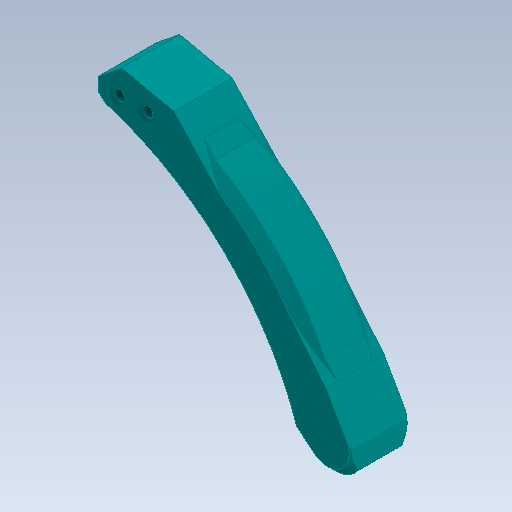
# Autodesk Inventor part: Tarsus
Saved by Autodesk Inventor 2020 (Build 240168000, 168)
## iProperties
Created: 2020-09-15
Part Number: Tarsus
Material: Generic
Document SubType Name: Modeling
Designer: Turing
Density: 1 g/cm^3
Appearance: Gray
Mass: 22.7557 g
Surface Area: 61.6652 cm^2
Volume: 22.7557 cm^3
Author: Turing
Autodesk Inventor part; units mm, degrees
ref_plane "YZ Plane" through (0, 0, 0) normal (1, 0, 0) x (0, 1, 0)
ref_plane "XZ Plane" through (0, 0, 0) normal (0, 1, 0) x (-1, 0, 0)
ref_plane "XY Plane" through (0, 0, 0) normal (0, 0, 1) x (1, 0, 0)
sketch "Sketch1" plane through (0, 0, 0) normal (0, 0, 1) x (1, 0, 0)
  circle A0 centre (0, 0) radius 1.5
  line L0 (0, 0) -> (8, 0)
  circle A1 centre (8, 0) radius 1.5
  line L1 (8, 0) -> (15.5, 0)
  line L2 (15.5, 0) -> (15.5, 4)
  line L3 (15.5, 0) -> (15.5, -4)
  line L4 (15.5, 4) -> (0.8426, 7.1878)
  line L5 (15.5, -4) -> (0.8886, -7.3921)
  line L6 (0, 0) -> (-8, 0)
  line L7 (0.8886, -7.3921) -> (-8, 0)
  line L8 (-8, 0) -> (0.8426, 7.1878)
  dimension "d0" = 3
  dimension "d1" = 8
  dimension "d2" = 3
  dimension "d3" = 7.5
  dimension "d4" = 4
  dimension "d5" = 4
  dimension "d6" = 102.27
  dimension "d7" = 103.07
  dimension "d8" = 15
  dimension "d9" = 15
  dimension "d10" = 8
  constraints: 18 end point, 3 horizontal, 2 centre point, 2 coincident, 2 vertical
  measures "d0" diameter of A0
  measures "d1" distance of L0.start L0.end
  measures "d2" diameter of A1
  measures "d3" distance of L1.start L1.end
  measures "d4" distance of L1.end L2.end
  measures "d5" distance of L1.end L3.end
  measures "d6" angle of L2 L4
  measures "d7" angle of L3 L5
  measures "d8" distance of L3.end L5.end
  measures "d9" distance of L2.end L4.end
  measures "d10" distance of L0.start L6.end
extrude "Extrusion1" add sketch "Sketch1" against normal blind 16.2 contours L0 A1 L1 L3 L5 L7 L6 A0 | A0 L6 L8 L4 L2 L1 A1 L0
sketch "Sketch2" plane through (0, 0, 0) normal (0, 0, 1) x (1, 0, 0)
  line L0 (15.5, 4) -> (0.8426, 7.1878) projected
  line L1 (0.8426, 7.1878) -> (-8, 0) projected
  line L2 (-8, 0) -> (0.8886, -7.3921) projected
  line L3 (0.8886, -7.3921) -> (15.5, -4) projected
  line L4 (15.5, -4) -> (15.5, 4) projected
  circle A0 centre (8, 0) radius 1.5 projected
  circle A1 centre (0, 0) radius 1.5 projected
  line L5 (0.8886, -7.3921) -> (7.7175, -14.6973)
  line L6 (15.5, 4) -> (22.3289, -3.3052)
  arc A2 (41.8621, -51.2233) -> (7.7175, -14.6973) centre (-26.8658, -81.248) ccw
  arc A3 (56.4735, -39.8312) -> (22.3289, -3.3052) centre (-12.2544, -69.8559) ccw
  line L7 (41.8621, -51.2233) -> (53.4151, -60.7903)
  arc A4 (53.4151, -60.7903) -> (63.4535, -48.3329) centre (58.5175, -54.6287) ccw
  line L8 (63.4535, -48.3329) -> (56.4735, -39.8312)
  dimension "d13" = 10
  dimension "d14" = 60
  dimension "d15" = 10
  dimension "d17" = 50
  dimension "d18" = 75
  dimension "d19" = 50
  dimension "d20" = 75
  dimension "d29" = 15
  dimension "d30" = 11
  dimension "d31" = 8
  dimension "d32" = 141.656
  constraints: 8 end point, 6 point on circle, 3 centre point, 2 point on line, 1 parallel, 1 tangent
  measures "d13" distance of L2.end L5.end
  measures "d14" angle of L3 L5
  measures "d15" distance of L0.start L6.end
  measures "d17" distance of L5.end L7.start
  measures "d18" radius of A2
  measures "d19" distance of L6.end L8.end
  measures "d20" radius of A3
  measures "d29" distance of L7.start L7.end
  measures "d30" distance of L8.end L8.start
  measures "d31" radius of A4
  measures "d32" angle of L0 L8
extrude "Extrusion2" add sketch "Sketch2" against normal up to surface (16.2 mm away) contours L6 A3 L8 A4 L7 A2 L5 L3 L4
chamfer "Chamfer2" distance 6 angle 45 2 edges at (27.9232, -30.0312, 0) (27.9232, -30.0312, -16.2)
chamfer "Chamfer3" distance 2.5 angle 45 4 edges at (42.5346, -18.6391, -16.2) (42.5346, -18.6391, 0) (22.3289, -3.3052, -8.1) (56.4735, -39.8312, -8.1)
chamfer "Chamfer4" distance 8.5 angle 45 1 edges at (63.4535, -48.3329, -8.1)
chamfer "Chamfer5" distance 2 angle 45 4 edges at (61.1284, -62.1906, 0) (52.1804, -59.7678, 0) (61.1284, -62.1906, -16.2) (52.1804, -59.7678, -16.2)
chamfer "Chamfer6" distance 3 angle 45 1 edges at (66.3346, -56.3297, -8.1)
chamfer "Chamfer7" distance 3 angle 45 1 edges at (-8, 0, -8.1)
body "Solid1"
